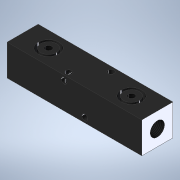
# Autodesk Inventor part: Manifold for gems solenoid valve vertical
Saved by Autodesk Inventor 2021.2 (Build 252289000, 289)
## iProperties
Created: 2021-03-30
Part Number: Manifold for gems solenoid valve vertical
Material: Aluminum 6061
Document SubType Name: Modeling
Designer: jl4459
Density: 2.7 g/cm^3
Appearance: Aluminum - Polished
Author: jl4459
Autodesk Inventor part; units mm, degrees
ref_plane "YZ Plane" through (0, 0, 0) normal (1, 0, 0) x (0, 1, 0)
ref_plane "XZ Plane" through (0, 0, 0) normal (0, 1, 0) x (-1, 0, 0)
ref_plane "XY Plane" through (0, 0, 0) normal (0, 0, 1) x (1, 0, 0)
sketch "Sketch1" plane through (0, 0, 0) normal (0, 0, 1) x (1, 0, 0)
  line L0 (-38.1, 9.525) -> (38.1, 9.525)
  line L1 (38.1, 9.525) -> (38.1, -9.525)
  line L2 (38.1, -9.525) -> (-38.1, -9.525)
  line L3 (-38.1, -9.525) -> (-38.1, 9.525)
  point P0 (0, 0)
  constraints: 8 end point, 2 parallel, 1 horizontal, 1 perpendicular
extrude "Extrusion1" add sketch "Sketch1" along normal blind 19.05
sketch "Sketch4" plane through (-38.1, 9.525, 0) normal (0, 1, 0) x (1, 0, 0)
  line L0 (76.2, -19.05) -> (0, -19.05) projected
  line L1 (76.2, 0) -> (76.2, -19.05) projected
  point P0 (38.1, 0)
  point P1 (63.5, -9.525)
  dimension "d34" = 9.525
  dimension "d35" = 12.7
  measures "d34" distance from line of L0 point (63.5, -9.525)
  measures "d35" distance from line of L1 point (63.5, -9.525)
hole "Hole3" at (25.4, 9.525, 9.525) direction (0, -1, 0) diameter 3.9624 depth 9.525 thread size "10-32 UNF" class "2B" standard "ANSI Unified Screw Threads"
sketch "Sketch5" plane through (-38.1, 9.525, 0) normal (0, 1, 0) x (1, 0, 0)
  line L0 (76.2, -19.05) -> (0, -19.05) projected
  line L1 (0, 0) -> (0, -19.05) projected
  point P0 (38.1, 0)
  point P1 (12.7, -9.525)
  dimension "d43" = 9.525
  dimension "d82" = 12.7
  measures "d43" distance from line of L0 point (12.7, -9.525)
  measures "d82" distance from line of L1 point (12.7, -9.525)
hole "Hole4" at (-25.4, 9.525, 9.525) direction (0, -1, 0) diameter 3.9624 depth 9.525 thread size "10-32 UNF" class "2B" standard "ANSI Unified Screw Threads"
sketch "Sketch6" plane through (-38.1, 9.525, 0) normal (0, 1, 0) x (1, 0, 0)
  line L0 (76.2, 0) -> (76.2, -19.05) projected
  line L1 (76.2, 0) -> (0, 0) projected
  point P0 (38.1, 0)
  point P1 (44.45, -2.9464)
  dimension "d51" = 31.75
  dimension "d52" = 2.9464
  measures "d51" distance from line of L0 point (44.45, -2.946)
  measures "d52" distance from line of L1 point (44.45, -2.946)
hole "Hole5" at (6.35, 9.525, 2.9464) direction (0, -1, 0) diameter 3.6576 end through all
sketch "Sketch7" plane through (-38.1, 9.525, 0) normal (0, 1, 0) x (1, 0, 0)
  line L0 (0, 0) -> (0, -19.05) projected
  line L1 (76.2, -19.05) -> (0, -19.05) projected
  point P0 (38.1, 0)
  point P1 (31.75, -16.1036)
  dimension "d60" = 31.75
  dimension "d61" = 2.9464
  measures "d60" distance from line of L0 point (31.75, -16.104)
  measures "d61" distance from line of L1 point (31.75, -16.104)
hole "Hole6" at (-6.35, 9.525, 16.1036) direction (0, -1, 0) diameter 3.6576 end through all
sketch "Sketch8" plane through (0, 0, 0) normal (0, 0, -1) x (-1, 0, 0)
  line L0 (-38.1, 9.525) -> (38.1, 9.525) projected
  line L1 (38.1, 9.525) -> (38.1, -9.525) projected
  line L2 (-38.1, -9.525) -> (-38.1, 9.525) projected
  line L3 (38.1, -9.525) -> (-38.1, -9.525) projected
  point P0 (0, 0)
  point P1 (6.35, 6.5786)
  point P2 (-6.35, -6.5786)
  dimension "d69" = 2.9464
  dimension "d70" = 31.75
  dimension "d71" = 31.75
  dimension "d72" = 2.9464
  measures "d69" distance from line of L0 point (6.35, 6.579)
  measures "d70" distance from line of L1 point (6.35, 6.579)
  measures "d71" distance from line of L2 point (-6.35, -6.579)
  measures "d72" distance from line of L3 point (-6.35, -6.579)
hole "Hole7" at (-6.35, 6.5786, 0) at (6.35, -6.5786, 0) direction (0, 0, 1) diameter 3.6576 end through all
sketch "Sketch9" plane through (-38.1, 9.525, 0) normal (0, 1, 0) x (1, 0, 0)
  circle A0 centre (63.5, -9.525) radius 1.9812 projected
  circle A1 centre (63.5, -9.525) radius 4.826
  circle A2 centre (63.5, -9.525) radius 6.35
  point P0 (38.1, 0)
  dimension "d83" = 9.652
  dimension "d84" = 12.7
  constraints: 2 centre point, 2 coincident
  measures "d83" diameter of A1
  measures "d84" diameter of A2
extrude "Extrusion2" cut sketch "Sketch9" against normal blind 5.08 contours A2
sketch "Sketch11" plane through (-38.1, 9.525, 0) normal (0, 1, 0) x (1, 0, 0)
  circle A0 centre (12.7, -9.525) radius 1.9812 projected
  circle A1 centre (12.7, -9.525) radius 4.826
  circle A2 centre (12.7, -9.525) radius 6.35
  point P0 (38.1, 0)
  dimension "d97" = 9.652
  dimension "d98" = 12.7
  constraints: 2 centre point, 2 coincident
  measures "d97" diameter of A1
  measures "d98" diameter of A2
extrude "Extrusion3" cut sketch "Sketch11" against normal blind 5.08 contours A2
sketch "Sketch13" plane through (-38.1, -9.525, 0) normal (0, -1, 0) x (1, 0, 0)
  line L0 (76.2, 0) -> (76.2, 19.05) projected
  line L1 (0, 19.05) -> (76.2, 19.05) projected
  point P0 (38.1, 0)
  point P1 (63.5, 15.113)
  dimension "d113" = 12.7
  dimension "d114" = 3.937
  measures "d113" distance from line of L0 point (63.5, 15.113)
  measures "d114" distance from line of L1 point (63.5, 15.113)
hole "Hole10" at (25.4, -9.525, 15.113) direction (0, 1, 0) diameter 1.5875 depth 14.2875
sketch "Sketch14" plane through (-38.1, -9.525, 0) normal (0, -1, 0) x (1, 0, 0)
  line L0 (0, 0) -> (0, 19.05) projected
  line L1 (0, 19.05) -> (76.2, 19.05) projected
  point P0 (38.1, 0)
  point P1 (12.7, 15.113)
  dimension "d122" = 12.7
  dimension "d123" = 3.937
  measures "d122" distance from line of L0 point (12.7, 15.113)
  measures "d123" distance from line of L1 point (12.7, 15.113)
hole "Hole11" at (-25.4, -9.525, 15.113) direction (0, 1, 0) diameter 1.5875 depth 14.2875
sketch "Sketch15" plane through (-38.1, -9.525, 0) normal (0, -1, 0) x (1, 0, 0)
  line L0 (76.2, 0) -> (76.2, 19.05) projected
  line L1 (0, 19.05) -> (76.2, 19.05) projected
  point P0 (38.1, 0)
  point P1 (63.5, 15.113)
  dimension "d131" = 12.7
  dimension "d132" = 3.937
  measures "d131" distance from line of L0 point (63.5, 15.113)
  measures "d132" distance from line of L1 point (63.5, 15.113)
hole "Hole12" at (25.4, -9.525, 15.113) direction (0, 1, 0) diameter 3.9624 depth 4.318 thread size "10-32 UNF" class "2B" standard "ANSI Unified Screw Threads"
sketch "Sketch16" plane through (-38.1, -9.525, 0) normal (0, -1, 0) x (1, 0, 0)
  line L0 (0, 0) -> (0, 19.05) projected
  line L1 (0, 19.05) -> (76.2, 19.05) projected
  point P0 (38.1, 0)
  point P1 (12.7, 15.113)
  dimension "d140" = 12.7
  dimension "d141" = 3.937
  measures "d140" distance from line of L0 point (12.7, 15.113)
  measures "d141" distance from line of L1 point (12.7, 15.113)
hole "Hole13" at (-25.4, -9.525, 15.113) direction (0, 1, 0) diameter 3.9624 depth 4.318 thread size "10-32 UNF" class "2B" standard "ANSI Unified Screw Threads"
move faces "Move5" translate (3.175, 0, 0) faces at (28.0866, -1.9767, 19.05) (38.1, -3.175, 6.35)
move faces "Move6" translate (-3.175, 0, 0) faces at (-38.1, 3.175, 6.35)
sketch "Sketch17" plane through (41.275, -9.525, 0) normal (1, 0, 0) x (0, 0, -1)
  line L0 (0, 19.05) -> (-19.05, 19.05) projected
  line L1 (0, 0) -> (0, 19.05) projected
  point P0 (0, 9.525)
  point P1 (-9.525, 9.525)
  dimension "d167" = 9.525
  dimension "d168" = 9.525
  measures "d167" distance from line of L0 point (-9.525, 9.525)
  measures "d168" distance from line of L1 point (-9.525, 9.525)
hole "Hole14" at (41.275, 0, 9.525) direction (-1, 0, 0) diameter 7.9502 depth 50.8 taper from width 8.7366 to width 8.304 over 6.924 thread size "1/8" designation "1/8 - 27 NPT" standard "NPT"
sketch "Sketch18" plane through (-41.275, -9.525, 0) normal (-1, 0, 0) x (0, 0, 1)
  line L0 (0, 19.05) -> (19.05, 19.05) projected
  line L1 (19.05, 19.05) -> (19.05, 0) projected
  point P0 (0, 9.525)
  point P1 (9.525, 9.525)
  dimension "d178" = 9.525
  dimension "d179" = 9.525
  measures "d178" distance from line of L0 point (9.525, 9.525)
  measures "d179" distance from line of L1 point (9.525, 9.525)
hole "Hole15" at (-41.275, 0, 9.525) direction (1, 0, 0) diameter 7.9502 depth 50.8 taper from width 8.7366 to width 8.304 over 6.924 thread size "1/8" designation "1/8 - 27 NPT" standard "NPT"
body "Solid1"
